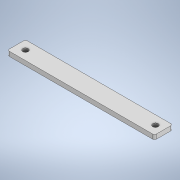
# Autodesk Inventor part: Slider_Winkel_Abstandshalter
Saved by Autodesk Inventor 2022.2 (Build 262287010, 287A)
## iProperties
Created: 2024-01-10
Part Number: Slider_Winkel_Abstandshalter
Material: Generisch
Document SubType Name: Modeling
Designer: ppovolni
Density: 1 g/cm^3
Appearance: Vorgabe
Author: ppovolni
Autodesk Inventor part; units mm, degrees
ref_plane "YZ Plane" through (0, 0, 0) normal (1, 0, 0) x (0, 1, 0)
ref_plane "XZ Plane" through (0, 0, 0) normal (0, 1, 0) x (-1, 0, 0)
ref_plane "XY Plane" through (0, 0, 0) normal (0, 0, 1) x (1, 0, 0)
sketch "Skizze1" plane through (0, 0, 0) normal (0, 1, 0) x (-1, 0, 0)
  line L0 (-2, 0) -> (-161.05, 0)
  line L1 (-163.05, -2) -> (-163.05, -18)
  line L2 (-161.05, -20) -> (-2, -20)
  line L3 (0, -18) -> (0, -2)
  circle A0 centre (-154.05, -10) radius 3.05
  line L4 (0, -10) -> (-163.05, -10) construction
  line L5 (-163.05, -20) -> (-164.05, -20) construction
  line L6 (-164.05, -20) -> (-164.05, -1) construction
  line L7 (-164.05, -1) -> (-163.05, -1) construction
  line L8 (-163.05, -1) -> (-163.05, -20) construction
  line L9 (-164.05, -20) -> (-169.05, -20) construction
  line L10 (-169.05, -20) -> (-169.05, -1) construction
  line L11 (-169.05, -1) -> (-164.05, -1) construction
  line L12 (-164.05, -1) -> (-164.05, -20) construction
  circle A1 centre (-10, -10) radius 3.05
  line L13 (-13.05, -20) -> (-13.05, 0) construction
  arc A2 (-2, -20) -> (0, -18) centre (-2, -18) ccw
  arc A3 (0, -2) -> (-2, 0) centre (-2, -2) ccw
  arc A4 (-163.05, -18) -> (-161.05, -20) centre (-161.05, -18) ccw
  arc A5 (-161.05, 0) -> (-163.05, -2) centre (-161.05, -2) ccw
  point P0 (0, 0)
  point P1 (0, -20)
  dimension "d0" = 20
  dimension "d2" = 5
  dimension "d3" = 1
  dimension "d5" = 10
  dimension "d6" = 6.1
  dimension "d7" = 156
  dimension "d8" = 10
  dimension "d9" = 6.1
  dimension "d10" = 2
  constraints: 28 end point, 11 point on line, 9 tangent, 8 point on circle, 6 centre point, 6 parallel, 4 perpendicular, 3 equal radius, 3 horizontal, 2 midpoint
  measures "d0" distance of point (0, -20) point (0, 0)
  measures "d2" distance of L5.end L9.end
  measures "d3" distance of L5.start L5.end
  measures "d5" distance from line of A0.centre L6
  measures "d6" diameter of A1
  measures "d7" distance between parallel lines of L10 L13
  measures "d8" distance from line of L3 A1.centre
  measures "d9" diameter of A0
  measures "d10" radius of A2
extrude "Extrusion1" add sketch "Skizze1" along normal blind 5
